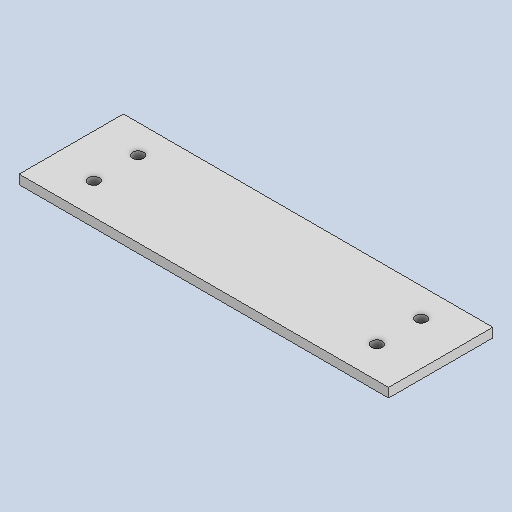
# Autodesk Inventor part: A-05
Saved by Autodesk Inventor 2023 (Build 270158000, 158)
## iProperties
Created: 2022-06-11
Part Number: A-05
Material: Generic
Document SubType Name: Modeling
Designer: kfcs7
Density: 1 g/cm^3
Appearance: Default
Author: kfcs7
Autodesk Inventor part; units mm, degrees
ref_plane "YZ Plane" through (0, 0, 0) normal (1, 0, 0) x (0, 1, 0)
ref_plane "XZ Plane" through (0, 0, 0) normal (0, 1, 0) x (-1, 0, 0)
ref_plane "XY Plane" through (0, 0, 0) normal (0, 0, 1) x (1, 0, 0)
sketch "Sketch2" plane through (0, 0, 0) normal (0, 1, 0) x (-1, 0, 0)
  line L0 (-48.208, 12.0672) -> (-48.208, 5.8672) construction
  line L1 (-48.208, 12.0672) -> (43.792, 12.0672) construction
  line L2 (43.792, 12.0672) -> (43.792, 5.8672) construction
  line L3 (37.542, 5.8672) -> (43.792, 5.8672) construction
  line L4 (37.542, 5.8672) -> (37.2414, 5.5672) construction
  line L5 (37.2414, 5.5672) -> (30.3425, 5.5672) construction
  line L6 (30.3425, 5.5672) -> (30.042, 5.8672) construction
  line L7 (-39.058, 5.8672) -> (30.042, 5.8672) construction
  line L8 (-39.058, 5.8672) -> (-39.3586, 5.5672) construction
  line L9 (-39.3586, 5.5672) -> (-46.2575, 5.5672) construction
  line L10 (-46.2575, 5.5672) -> (-46.558, 5.8672) construction
  line L11 (-48.208, 5.8672) -> (-46.558, 5.8672) construction
  circle A0 centre (-42.808, 8.5672) radius 1.25 construction
  circle A1 centre (33.792, 8.5672) radius 1.25 construction
  circle A2 centre (33.792, 8.5672) radius 1.5
  circle A3 centre (-42.808, 8.5672) radius 1.5
  line L12 (45.492, 29.0672) -> (-54.508, 29.0672)
  line L13 (-54.508, 29.0672) -> (-54.508, 0.8672)
  line L14 (-54.508, 0.8672) -> (45.492, 0.8672)
  line L15 (45.492, 0.8672) -> (45.492, 29.0672)
  line L16 (-42.808, 8.5672) -> (33.792, 8.5672) construction
  line L17 (-4.508, 8.5672) -> (-4.508, 29.0672) construction
  line L18 (-48.208, 24.0672) -> (-48.208, 17.8672) construction
  line L19 (-48.208, 24.0672) -> (43.792, 24.0672) construction
  line L20 (43.792, 24.0672) -> (43.792, 17.8672) construction
  line L21 (37.542, 17.8672) -> (43.792, 17.8672) construction
  line L22 (37.542, 17.8672) -> (37.2414, 17.5672) construction
  line L23 (37.2414, 17.5672) -> (30.3425, 17.5672) construction
  line L24 (30.3425, 17.5672) -> (30.042, 17.8672) construction
  line L25 (-39.058, 17.8672) -> (30.042, 17.8672) construction
  line L26 (-39.058, 17.8672) -> (-39.3586, 17.5672) construction
  line L27 (-39.3586, 17.5672) -> (-46.2575, 17.5672) construction
  line L28 (-46.2575, 17.5672) -> (-46.558, 17.8672) construction
  line L29 (-48.208, 17.8672) -> (-46.558, 17.8672) construction
  circle A4 centre (-42.808, 20.5672) radius 1.25 construction
  circle A5 centre (33.792, 20.5672) radius 1.25 construction
  circle A6 centre (33.792, 20.5672) radius 1.5
  circle A7 centre (-42.808, 20.5672) radius 1.5
  point P0 (0, 0)
  dimension "d0" = 3
  dimension "d1" = 3
  dimension "d2" = 76.6
  dimension "d3" = 100
  dimension "d4" = 3
  dimension "d5" = 3
  dimension "d6" = 5
  dimension "d7" = 5
  constraints: 12 end point, 4 centre point, 4 coincident, 2 midpoint, 2 parallel, 2 perpendicular, 1 horizontal
  measures "d0" diameter of A2
  measures "d1" diameter of A3
  measures "d2" distance of L16.start L16.end
  measures "d3" distance of L12.start L12.end
  measures "d4" diameter of A6
  measures "d5" diameter of A7
  measures "d6" distance between parallel lines of L19 L12
  measures "d7" distance between parallel lines of L7 L14
extrude "Extrusion1" add sketch "Sketch2" along normal blind 2.5
equation "\"d1\" = d0"
equation "\"d4\" = d0"
equation "\"d5\" = d4"
equation "\"d7\" = d6"
body "Solid1"
